Autodesk Inventor part; units mm, degrees
(part 2 of 2)
  line L334 (130.81, 94.488) -> (130.81, 96.012) construction
  arc A396 (131.191, 96.012) -> (130.429, 96.012) centre (130.81, 96.012) ccw construction
  arc A397 (130.429, 94.488) -> (131.191, 94.488) centre (130.81, 94.488) ccw construction
  line L335 (133.35, 94.488) -> (133.35, 96.012) construction
  arc A398 (133.731, 96.012) -> (132.969, 96.012) centre (133.35, 96.012) ccw construction
  arc A399 (132.969, 94.488) -> (133.731, 94.488) centre (133.35, 94.488) ccw construction
  line L336 (133.35, 94.488) -> (133.35, 96.012) construction
  arc A400 (133.731, 96.012) -> (132.969, 96.012) centre (133.35, 96.012) ccw construction
  arc A401 (132.969, 94.488) -> (133.731, 94.488) centre (133.35, 94.488) ccw construction
  line L337 (135.89, 94.488) -> (135.89, 96.012) construction
  arc A402 (136.271, 96.012) -> (135.509, 96.012) centre (135.89, 96.012) ccw construction
  arc A403 (135.509, 94.488) -> (136.271, 94.488) centre (135.89, 94.488) ccw construction
  line L338 (135.89, 94.488) -> (135.89, 96.012) construction
  arc A404 (136.271, 96.012) -> (135.509, 96.012) centre (135.89, 96.012) ccw construction
  arc A405 (135.509, 94.488) -> (136.271, 94.488) centre (135.89, 94.488) ccw construction
  line L339 (138.43, 94.488) -> (138.43, 96.012) construction
  arc A406 (138.811, 96.012) -> (138.049, 96.012) centre (138.43, 96.012) ccw construction
  arc A407 (138.049, 94.488) -> (138.811, 94.488) centre (138.43, 94.488) ccw construction
  line L340 (138.43, 94.488) -> (138.43, 96.012) construction
  arc A408 (138.811, 96.012) -> (138.049, 96.012) centre (138.43, 96.012) ccw construction
  arc A409 (138.049, 94.488) -> (138.811, 94.488) centre (138.43, 94.488) ccw construction
  line L341 (140.97, 94.488) -> (140.97, 96.012) construction
  arc A410 (141.351, 96.012) -> (140.589, 96.012) centre (140.97, 96.012) ccw construction
  arc A411 (140.589, 94.488) -> (141.351, 94.488) centre (140.97, 94.488) ccw construction
  line L342 (140.97, 94.488) -> (140.97, 96.012) construction
  arc A412 (141.351, 96.012) -> (140.589, 96.012) centre (140.97, 96.012) ccw construction
  arc A413 (140.589, 94.488) -> (141.351, 94.488) centre (140.97, 94.488) ccw construction
  line L343 (143.51, 94.488) -> (143.51, 96.012) construction
  arc A414 (143.891, 96.012) -> (143.129, 96.012) centre (143.51, 96.012) ccw construction
  arc A415 (143.129, 94.488) -> (143.891, 94.488) centre (143.51, 94.488) ccw construction
  line L344 (143.51, 94.488) -> (143.51, 96.012) construction
  arc A416 (143.891, 96.012) -> (143.129, 96.012) centre (143.51, 96.012) ccw construction
  arc A417 (143.129, 94.488) -> (143.891, 94.488) centre (143.51, 94.488) ccw construction
  line L345 (39.1668, 91.1606) -> (40.6908, 91.1606) construction
  arc A418 (40.6908, 90.7796) -> (40.6908, 91.5416) centre (40.6908, 91.1606) ccw construction
  arc A419 (39.1668, 91.5416) -> (39.1668, 90.7796) centre (39.1668, 91.1606) ccw construction
  line L346 (39.1668, 91.1606) -> (40.6908, 91.1606) construction
  arc A420 (40.6908, 90.7796) -> (40.6908, 91.5416) centre (40.6908, 91.1606) ccw construction
  arc A421 (39.1668, 91.5416) -> (39.1668, 90.7796) centre (39.1668, 91.1606) ccw construction
  line L347 (45.6692, 91.1606) -> (47.1932, 91.1606) construction
  arc A422 (47.1932, 90.7796) -> (47.1932, 91.5416) centre (47.1932, 91.1606) ccw construction
  arc A423 (45.6692, 91.5416) -> (45.6692, 90.7796) centre (45.6692, 91.1606) ccw construction
  line L348 (45.6692, 91.1606) -> (47.1932, 91.1606) construction
  arc A424 (47.1932, 90.7796) -> (47.1932, 91.5416) centre (47.1932, 91.1606) ccw construction
  arc A425 (45.6692, 91.5416) -> (45.6692, 90.7796) centre (45.6692, 91.1606) ccw construction
  line L349 (39.1668, 86.6394) -> (40.6908, 86.6394) construction
  arc A426 (40.6908, 86.2584) -> (40.6908, 87.0204) centre (40.6908, 86.6394) ccw construction
  arc A427 (39.1668, 87.0204) -> (39.1668, 86.2584) centre (39.1668, 86.6394) ccw construction
  line L350 (39.1668, 86.6394) -> (40.6908, 86.6394) construction
  arc A428 (40.6908, 86.2584) -> (40.6908, 87.0204) centre (40.6908, 86.6394) ccw construction
  arc A429 (39.1668, 87.0204) -> (39.1668, 86.2584) centre (39.1668, 86.6394) ccw construction
  line L351 (45.6692, 86.6394) -> (47.1932, 86.6394) construction
  arc A430 (47.1932, 86.2584) -> (47.1932, 87.0204) centre (47.1932, 86.6394) ccw construction
  arc A431 (45.6692, 87.0204) -> (45.6692, 86.2584) centre (45.6692, 86.6394) ccw construction
  line L352 (45.6692, 86.6394) -> (47.1932, 86.6394) construction
  arc A432 (47.1932, 86.2584) -> (47.1932, 87.0204) centre (47.1932, 86.6394) ccw construction
  arc A433 (45.6692, 87.0204) -> (45.6692, 86.2584) centre (45.6692, 86.6394) ccw construction
  line L353 (62.0268, 91.1606) -> (63.5508, 91.1606) construction
  arc A434 (63.5508, 90.7796) -> (63.5508, 91.5416) centre (63.5508, 91.1606) ccw construction
  arc A435 (62.0268, 91.5416) -> (62.0268, 90.7796) centre (62.0268, 91.1606) ccw construction
  line L354 (62.0268, 91.1606) -> (63.5508, 91.1606) construction
  arc A436 (63.5508, 90.7796) -> (63.5508, 91.5416) centre (63.5508, 91.1606) ccw construction
  arc A437 (62.0268, 91.5416) -> (62.0268, 90.7796) centre (62.0268, 91.1606) ccw construction
  line L355 (68.5292, 91.1606) -> (70.0532, 91.1606) construction
  arc A438 (70.0532, 90.7796) -> (70.0532, 91.5416) centre (70.0532, 91.1606) ccw construction
  arc A439 (68.5292, 91.5416) -> (68.5292, 90.7796) centre (68.5292, 91.1606) ccw construction
  line L356 (68.5292, 91.1606) -> (70.0532, 91.1606) construction
  arc A440 (70.0532, 90.7796) -> (70.0532, 91.5416) centre (70.0532, 91.1606) ccw construction
  arc A441 (68.5292, 91.5416) -> (68.5292, 90.7796) centre (68.5292, 91.1606) ccw construction
  line L357 (62.0268, 86.6394) -> (63.5508, 86.6394) construction
  arc A442 (63.5508, 86.2584) -> (63.5508, 87.0204) centre (63.5508, 86.6394) ccw construction
  arc A443 (62.0268, 87.0204) -> (62.0268, 86.2584) centre (62.0268, 86.6394) ccw construction
  line L358 (62.0268, 86.6394) -> (63.5508, 86.6394) construction
  arc A444 (63.5508, 86.2584) -> (63.5508, 87.0204) centre (63.5508, 86.6394) ccw construction
  arc A445 (62.0268, 87.0204) -> (62.0268, 86.2584) centre (62.0268, 86.6394) ccw construction
  line L359 (68.5292, 86.6394) -> (70.0532, 86.6394) construction
  arc A446 (70.0532, 86.2584) -> (70.0532, 87.0204) centre (70.0532, 86.6394) ccw construction
  arc A447 (68.5292, 87.0204) -> (68.5292, 86.2584) centre (68.5292, 86.6394) ccw construction
  line L360 (68.5292, 86.6394) -> (70.0532, 86.6394) construction
  arc A448 (70.0532, 86.2584) -> (70.0532, 87.0204) centre (70.0532, 86.6394) ccw construction
  arc A449 (68.5292, 87.0204) -> (68.5292, 86.2584) centre (68.5292, 86.6394) ccw construction
  line L361 (88.6968, 91.1606) -> (90.2208, 91.1606) construction
  arc A450 (90.2208, 90.7796) -> (90.2208, 91.5416) centre (90.2208, 91.1606) ccw construction
  arc A451 (88.6968, 91.5416) -> (88.6968, 90.7796) centre (88.6968, 91.1606) ccw construction
  line L362 (88.6968, 91.1606) -> (90.2208, 91.1606) construction
  arc A452 (90.2208, 90.7796) -> (90.2208, 91.5416) centre (90.2208, 91.1606) ccw construction
  arc A453 (88.6968, 91.5416) -> (88.6968, 90.7796) centre (88.6968, 91.1606) ccw construction
  line L363 (95.1992, 91.1606) -> (96.7232, 91.1606) construction
  arc A454 (96.7232, 90.7796) -> (96.7232, 91.5416) centre (96.7232, 91.1606) ccw construction
  arc A455 (95.1992, 91.5416) -> (95.1992, 90.7796) centre (95.1992, 91.1606) ccw construction
  line L364 (95.1992, 91.1606) -> (96.7232, 91.1606) construction
  arc A456 (96.7232, 90.7796) -> (96.7232, 91.5416) centre (96.7232, 91.1606) ccw construction
  arc A457 (95.1992, 91.5416) -> (95.1992, 90.7796) centre (95.1992, 91.1606) ccw construction
  line L365 (88.6968, 86.6394) -> (90.2208, 86.6394) construction
  arc A458 (90.2208, 86.2584) -> (90.2208, 87.0204) centre (90.2208, 86.6394) ccw construction
  arc A459 (88.6968, 87.0204) -> (88.6968, 86.2584) centre (88.6968, 86.6394) ccw construction
  line L366 (88.6968, 86.6394) -> (90.2208, 86.6394) construction
  arc A460 (90.2208, 86.2584) -> (90.2208, 87.0204) centre (90.2208, 86.6394) ccw construction
  arc A461 (88.6968, 87.0204) -> (88.6968, 86.2584) centre (88.6968, 86.6394) ccw construction
  line L367 (95.1992, 86.6394) -> (96.7232, 86.6394) construction
  arc A462 (96.7232, 86.2584) -> (96.7232, 87.0204) centre (96.7232, 86.6394) ccw construction
  arc A463 (95.1992, 87.0204) -> (95.1992, 86.2584) centre (95.1992, 86.6394) ccw construction
  line L368 (95.1992, 86.6394) -> (96.7232, 86.6394) construction
  arc A464 (96.7232, 86.2584) -> (96.7232, 87.0204) centre (96.7232, 86.6394) ccw construction
  arc A465 (95.1992, 87.0204) -> (95.1992, 86.2584) centre (95.1992, 86.6394) ccw construction
  line L369 (112.8268, 91.1606) -> (114.3508, 91.1606) construction
  arc A466 (114.3508, 90.7796) -> (114.3508, 91.5416) centre (114.3508, 91.1606) ccw construction
  arc A467 (112.8268, 91.5416) -> (112.8268, 90.7796) centre (112.8268, 91.1606) ccw construction
  line L370 (112.8268, 91.1606) -> (114.3508, 91.1606) construction
  arc A468 (114.3508, 90.7796) -> (114.3508, 91.5416) centre (114.3508, 91.1606) ccw construction
  arc A469 (112.8268, 91.5416) -> (112.8268, 90.7796) centre (112.8268, 91.1606) ccw construction
  line L371 (119.3292, 91.1606) -> (120.8532, 91.1606) construction
  arc A470 (120.8532, 90.7796) -> (120.8532, 91.5416) centre (120.8532, 91.1606) ccw construction
  arc A471 (119.3292, 91.5416) -> (119.3292, 90.7796) centre (119.3292, 91.1606) ccw construction
  line L372 (119.3292, 91.1606) -> (120.8532, 91.1606) construction
  arc A472 (120.8532, 90.7796) -> (120.8532, 91.5416) centre (120.8532, 91.1606) ccw construction
  arc A473 (119.3292, 91.5416) -> (119.3292, 90.7796) centre (119.3292, 91.1606) ccw construction
  line L373 (112.8268, 86.6394) -> (114.3508, 86.6394) construction
  arc A474 (114.3508, 86.2584) -> (114.3508, 87.0204) centre (114.3508, 86.6394) ccw construction
  arc A475 (112.8268, 87.0204) -> (112.8268, 86.2584) centre (112.8268, 86.6394) ccw construction
  line L374 (112.8268, 86.6394) -> (114.3508, 86.6394) construction
  arc A476 (114.3508, 86.2584) -> (114.3508, 87.0204) centre (114.3508, 86.6394) ccw construction
  arc A477 (112.8268, 87.0204) -> (112.8268, 86.2584) centre (112.8268, 86.6394) ccw construction
  line L375 (119.3292, 86.6394) -> (120.8532, 86.6394) construction
  arc A478 (120.8532, 86.2584) -> (120.8532, 87.0204) centre (120.8532, 86.6394) ccw construction
  arc A479 (119.3292, 87.0204) -> (119.3292, 86.2584) centre (119.3292, 86.6394) ccw construction
  line L376 (119.3292, 86.6394) -> (120.8532, 86.6394) construction
  arc A480 (120.8532, 86.2584) -> (120.8532, 87.0204) centre (120.8532, 86.6394) ccw construction
  arc A481 (119.3292, 87.0204) -> (119.3292, 86.2584) centre (119.3292, 86.6394) ccw construction
  arc A482 (111.8616, 92.4701) -> (111.8616, 92.8483) centre (111.8616, 92.6592) ccw construction
  arc A483 (111.8616, 92.8483) -> (111.8616, 92.4701) centre (111.8616, 92.6592) ccw construction
  arc A484 (111.8616, 92.4701) -> (111.8616, 92.8483) centre (111.8616, 92.6592) ccw construction
  arc A485 (111.8616, 92.8483) -> (111.8616, 92.4701) centre (111.8616, 92.6592) ccw construction
  arc A486 (109.728, 58.9421) -> (109.728, 59.3203) centre (109.728, 59.1312) ccw
  arc A487 (109.728, 59.3203) -> (109.728, 58.9421) centre (109.728, 59.1312) ccw
  arc A488 (109.728, 58.9421) -> (109.728, 59.3203) centre (109.728, 59.1312) ccw
  arc A489 (109.728, 59.3203) -> (109.728, 58.9421) centre (109.728, 59.1312) ccw
  arc A490 (99.06, 76.9253) -> (99.06, 77.3035) centre (99.06, 77.1144) ccw
  arc A491 (99.06, 77.3035) -> (99.06, 76.9253) centre (99.06, 77.1144) ccw
  arc A492 (99.06, 76.9253) -> (99.06, 77.3035) centre (99.06, 77.1144) ccw
  arc A493 (99.06, 77.3035) -> (99.06, 76.9253) centre (99.06, 77.1144) ccw
  arc A494 (79.0956, 56.0465) -> (79.0956, 56.4247) centre (79.0956, 56.2356) ccw
  arc A495 (79.0956, 56.4247) -> (79.0956, 56.0465) centre (79.0956, 56.2356) ccw
  arc A496 (79.0956, 56.0465) -> (79.0956, 56.4247) centre (79.0956, 56.2356) ccw
  arc A497 (79.0956, 56.4247) -> (79.0956, 56.0465) centre (79.0956, 56.2356) ccw
  arc A498 (72.2376, 47.5121) -> (72.2376, 47.8903) centre (72.2376, 47.7012) ccw
  arc A499 (72.2376, 47.8903) -> (72.2376, 47.5121) centre (72.2376, 47.7012) ccw
  arc A500 (72.2376, 47.5121) -> (72.2376, 47.8903) centre (72.2376, 47.7012) ccw
  arc A501 (72.2376, 47.8903) -> (72.2376, 47.5121) centre (72.2376, 47.7012) ccw
  arc A502 (72.2376, 48.4265) -> (72.2376, 48.8047) centre (72.2376, 48.6156) ccw
  arc A503 (72.2376, 48.8047) -> (72.2376, 48.4265) centre (72.2376, 48.6156) ccw
  arc A504 (72.2376, 48.4265) -> (72.2376, 48.8047) centre (72.2376, 48.6156) ccw
  arc A505 (72.2376, 48.8047) -> (72.2376, 48.4265) centre (72.2376, 48.6156) ccw
  arc A506 (79.0956, 78.9065) -> (79.0956, 79.2847) centre (79.0956, 79.0956) ccw
  arc A507 (79.0956, 79.2847) -> (79.0956, 78.9065) centre (79.0956, 79.0956) ccw
  arc A508 (79.0956, 78.9065) -> (79.0956, 79.2847) centre (79.0956, 79.0956) ccw
  arc A509 (79.0956, 79.2847) -> (79.0956, 78.9065) centre (79.0956, 79.0956) ccw
  arc A510 (28.4988, 90.7937) -> (28.4988, 91.1719) centre (28.4988, 90.9828) ccw
  arc A511 (28.4988, 91.1719) -> (28.4988, 90.7937) centre (28.4988, 90.9828) ccw
  arc A512 (28.4988, 90.7937) -> (28.4988, 91.1719) centre (28.4988, 90.9828) ccw
  arc A513 (28.4988, 91.1719) -> (28.4988, 90.7937) centre (28.4988, 90.9828) ccw
  arc A514 (32.6136, 90.7937) -> (32.6136, 91.1719) centre (32.6136, 90.9828) ccw
  arc A515 (32.6136, 91.1719) -> (32.6136, 90.7937) centre (32.6136, 90.9828) ccw
  arc A516 (32.6136, 90.7937) -> (32.6136, 91.1719) centre (32.6136, 90.9828) ccw
  arc A517 (32.6136, 91.1719) -> (32.6136, 90.7937) centre (32.6136, 90.9828) ccw
  arc A518 (23.622, 88.8125) -> (23.622, 89.1907) centre (23.622, 89.0016) ccw
  arc A519 (23.622, 89.1907) -> (23.622, 88.8125) centre (23.622, 89.0016) ccw
  arc A520 (23.622, 88.8125) -> (23.622, 89.1907) centre (23.622, 89.0016) ccw
  arc A521 (23.622, 89.1907) -> (23.622, 88.8125) centre (23.622, 89.0016) ccw
  point P0 (0, 0)
  constraints: 912 point on circle, 754 end point, 522 centre point
extrude "押し出し1" add sketch "スケッチ1" along normal blind 1.6 contours L4 A6 A8 L3 L2 L6 A10 A12 L5 L1 L10 A29 A21 L14 A35 A28 A33 A26 A34 L13 A18 A27 L9 A23 A19 L11 A32 A22 A30 L12 A16 A25 L8 L0 | L4 L3 A8 A6 | A25 A16 L12 L8 | A22 A32 L11 A30 | L6 L5 A12 A10 | A19 A23 L9 L11 | A27 A18 L13 L9 | A34 A26 A33 L13 | A28 A35 L14 A33 | L10 L14 A21 A29 picked at (11.1748, 76.8697) picked at (67.0978, -7.475) picked at (147.9841, 76.8715) picked at (92.0611, -7.4751) picked at (99.0256, -7.475)
